J2 (Autodesk Fusion 360 design; units mm, degrees)
part number: 2026-05-30-23-24-39-589
Autodesk Fusion 360 part; units mm, degrees
sketch "Sketch1" plane through (0, 0, 0) normal (0, 0, 1) x (1, 0, 0)
  circle A0 centre (0, 0) radius 3.5
  dimension "d1" = 7
  constraint coincident A0.centre origin
  measures "d1" diameter of A0
extrude "Extrude1" add sketch "Sketch1" along normal blind 10
sketch "Sketch2" plane through (0, 0, 10) normal (0, 0, 1) x (-1, 0, 0)
  circle A0 centre (0, 0) radius 3.5
  line L0 (-1, 3) -> (1, 3)
  line L1 (1, -3) -> (-1, -3)
  line L2 (-3, 1) -> (-3, -1)
  line L3 (3, -1) -> (3, 1)
  line L4 (1, 3) -> (1, 1)
  line L5 (1, -1) -> (1, -3)
  line L6 (-3, -1) -> (-1, -1)
  line L7 (1, -1) -> (3, -1)
  line L8 (-1, -3) -> (-1, -1)
  line L9 (-1, 1) -> (-1, 3)
  line L10 (3, 1) -> (1, 1)
  line L11 (-1, 1) -> (-3, 1)
  dimension "d4" = 2
  dimension "d5" = 6
  dimension "d6" = 6
  constraint horizontal L0
  constraint vertical L4
  constraint horizontal L1
  constraint vertical L8
  constraint horizontal L10
  constraint vertical L2
  constraint horizontal L6
  constraint vertical L3
  constraint collinear L4 L5
  constraint collinear L6 L7
  constraint collinear L8 L9
  constraint collinear L10 L11
  measures "d4" distance of L0.start L0.end
  measures "d5" distance of L0.start L1.end
  measures "d6" distance of L3.end L2.start
extrude "Extrude2" cut sketch "Sketch2" against normal blind 10 contours L0 L1 L2 L3 L4 L5 L6 L7 L8 L9 L10 L11
